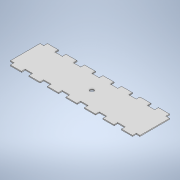
# Autodesk Inventor part: BridgeBottom
Saved by Autodesk Inventor 2022 (Build 260153000, 153)
## iProperties
Created: 2022-03-02
Part Number: BridgeBottom
Material: Generic
Document SubType Name: Modeling
Designer: anjarwala7025
Density: 1 g/cm^3
Appearance: Default
Author: anjarwala7025
Autodesk Inventor part; units mm, degrees
ref_plane "YZ Plane" through (0, 0, 0) normal (1, 0, 0) x (0, 1, 0)
ref_plane "XZ Plane" through (0, 0, 0) normal (0, 1, 0) x (-1, 0, 0)
ref_plane "XY Plane" through (0, 0, 0) normal (0, 0, 1) x (1, 0, 0)
sketch "Sketch1" plane through (0, 0, 0) normal (0, 1, 0) x (-1, 0, 0)
  line L0 (0, 0) -> (-444.5, 0)
  line L1 (-444.5, 0) -> (-444.5, -127)
  line L2 (-444.5, -127) -> (0, -127)
  line L3 (0, -127) -> (0, 0)
  dimension "d0" = 444.5
  dimension "d1" = 127
  constraints: 8 end point, 2 parallel, 1 horizontal, 1 perpendicular
  measures "d0" distance of L2.end L1.end
  measures "d1" distance of L1.end L0.end
extrude "Extrusion1" add sketch "Sketch1" along normal blind 3.175
sketch "Sketch2" plane through (0, 3.175, 0) normal (0, 1, 0) x (1, 0, 0)
  line L0 (0, 127) -> (0, 0) projected
  line L1 (0, 114.3) -> (12.7, 114.3)
  line L2 (12.7, 114.3) -> (12.7, 127)
  line L3 (444.5, 127) -> (0, 127) projected
  line L4 (50.8, 127) -> (50.8, 114.3)
  line L5 (50.8, 114.3) -> (76.2, 114.3)
  line L6 (76.2, 114.3) -> (76.2, 127)
  line L7 (114.3, 127) -> (114.3, 114.3)
  line L8 (114.3, 114.3) -> (139.7, 114.3)
  line L9 (139.7, 114.3) -> (139.7, 127)
  line L10 (177.8, 127) -> (177.8, 114.3)
  line L11 (177.8, 114.3) -> (203.2, 114.3)
  line L12 (203.2, 114.3) -> (203.2, 127)
  line L13 (241.3, 127) -> (241.3, 114.3)
  line L14 (241.3, 114.3) -> (266.7, 114.3)
  line L15 (266.7, 114.3) -> (266.7, 127)
  line L16 (304.8, 127) -> (304.8, 114.3)
  line L17 (304.8, 114.3) -> (330.2, 114.3)
  line L18 (330.2, 114.3) -> (330.2, 127)
  line L19 (368.3, 127) -> (368.3, 114.3)
  line L20 (368.3, 114.3) -> (393.7, 114.3)
  line L21 (393.7, 114.3) -> (393.7, 127)
  line L22 (431.8, 127) -> (431.8, 114.3)
  line L23 (431.8, 114.3) -> (444.5, 114.3)
  line L24 (444.5, 0) -> (444.5, 127) projected
  line L25 (0, 114.3) -> (0, 127)
  line L26 (50.8, 127) -> (76.2, 127)
  line L27 (114.3, 127) -> (139.7, 127)
  line L28 (177.8, 127) -> (203.2, 127)
  line L29 (241.3, 127) -> (266.7, 127)
  line L30 (304.8, 127) -> (330.2, 127)
  line L31 (368.3, 127) -> (393.7, 127)
  line L32 (431.8, 127) -> (444.5, 127)
  line L33 (0, 127) -> (12.7, 127)
  point P0 (444.5, 114.3)
  point P1 (12.7, 127)
  dimension "d4" = 12.7
  dimension "d6" = 12.7
  dimension "d7" = 12.7
  dimension "d8" = 12.7
  dimension "d9" = 25.4
  dimension "d10" = 38.1
  dimension "d11" = 25.4
  dimension "d12" = 38.1
  dimension "d13" = 25.4
  dimension "d14" = 38.1
  dimension "d15" = 25.4
  dimension "d16" = 38.1
  dimension "d17" = 25.4
  dimension "d18" = 38.1
  dimension "d19" = 25.4
  dimension "d20" = 38.1
  dimension "d22" = 0
  dimension "d42" = 12.7
  dimension "d53" = 38.1
  constraints: 62 end point, 13 vertical, 9 perpendicular, 7 horizontal, 1 collinear, 1 point on line, 14 other
  measures "d4" distance of L1.start L1.end
  measures "d6" length of L1
  measures "d7" distance of L1.end L2.end
  measures "d8" distance of L4.start L4.end
  measures "d9" distance of L4.end L5.end
  measures "d10" distance between parallel lines of L4 L2
  measures "d11" distance of L7.end L8.end
  measures "d12" distance between parallel lines of L7 L6
  measures "d13" distance of L10.end L11.end
  measures "d14" distance between parallel lines of L10 L9
  measures "d15" distance of L13.end L14.end
  measures "d16" distance between parallel lines of L13 L12
  measures "d17" distance of L16.end L17.end
  measures "d18" distance between parallel lines of L16 L15
  measures "d19" distance of L19.end L20.end
  measures "d20" distance between parallel lines of L19 L18
  measures "d22" distance from line of L24 L23.end
  measures "d42" distance of L22.start L22.end
  measures "d53" distance between parallel lines of L22 L21
extrude "Extrusion2" cut sketch "Sketch2" against normal through all
sketch "Sketch3" plane through (0, 3.175, 0) normal (0, 1, 0) x (1, 0, 0)
  line L0 (0, 0) -> (444.5, 0) projected
  line L1 (0, 0) -> (12.7, 0)
  line L2 (12.7, 0) -> (12.7, 12.7)
  line L3 (12.7, 12.7) -> (0, 12.7)
  line L4 (0, 12.7) -> (0, 0)
  line L5 (50.8, 0) -> (76.2, 0)
  line L6 (76.2, 0) -> (76.2, 12.7)
  line L7 (76.2, 12.7) -> (50.8, 12.7)
  line L8 (50.8, 12.7) -> (50.8, 0)
  line L9 (114.3, 0) -> (139.7, 0)
  line L10 (139.7, 0) -> (139.7, 12.7)
  line L11 (139.7, 12.7) -> (114.3, 12.7)
  line L12 (114.3, 12.7) -> (114.3, 0)
  line L13 (177.8, 0) -> (203.2, 0)
  line L14 (203.2, 0) -> (203.2, 12.7)
  line L15 (203.2, 12.7) -> (177.8, 12.7)
  line L16 (177.8, 12.7) -> (177.8, 0)
  line L17 (241.3, 0) -> (266.7, 0)
  line L18 (266.7, 0) -> (266.7, 12.7)
  line L19 (266.7, 12.7) -> (241.3, 12.7)
  line L20 (241.3, 12.7) -> (241.3, 0)
  line L21 (304.8, 0) -> (330.2, 0)
  line L22 (330.2, 0) -> (330.2, 12.7)
  line L23 (330.2, 12.7) -> (304.8, 12.7)
  line L24 (304.8, 12.7) -> (304.8, 0)
  line L25 (368.3, 0) -> (393.7, 0)
  line L26 (393.7, 0) -> (393.7, 12.7)
  line L27 (393.7, 12.7) -> (368.3, 12.7)
  line L28 (368.3, 12.7) -> (368.3, 0)
  line L29 (444.5, 0) -> (444.5, 114.3) projected
  line L30 (444.5, 0) -> (431.8, 0)
  line L31 (431.8, 0) -> (431.8, 12.7)
  line L32 (431.8, 12.7) -> (444.5, 12.7)
  line L33 (444.5, 12.7) -> (444.5, 0)
  point P0 (431.8, 0)
  point P1 (393.7, 0)
  point P2 (330.2, 0)
  point P3 (266.7, 0)
  point P4 (203.2, 0)
  point P5 (139.7, 0)
  point P6 (50.8, 0)
  point P7 (76.2, 0)
  point P8 (12.7, 0)
  dimension "d25" = 12.7
  dimension "d26" = 12.7
  dimension "d27" = 25.4
  dimension "d28" = 38.1
  dimension "d29" = 25.4
  dimension "d30" = 25.4
  dimension "d31" = 25.4
  dimension "d32" = 25.4
  dimension "d33" = 25.4
  dimension "d34" = 12.7
  dimension "d35" = 38.1
  dimension "d36" = 38.1
  dimension "d37" = 38.1
  dimension "d38" = 38.1
  dimension "d39" = 38.1
  constraints: 64 end point, 16 parallel, 11 point on line, 8 horizontal, 8 perpendicular
  measures "d25" distance of L3.end L2.end
  measures "d26" distance of L2.end L1.end
  measures "d27" distance of L7.end L6.end
  measures "d28" distance between parallel lines of L8 L2
  measures "d29" distance of L11.end L10.end
  measures "d30" distance of L15.end L14.end
  measures "d31" distance of L19.end L18.end
  measures "d32" distance of L23.end L22.end
  measures "d33" distance of L27.end L26.end
  measures "d34" distance of L31.end L32.end
  measures "d35" distance between parallel lines of L12 L6
  measures "d36" distance between parallel lines of L16 L10
  measures "d37" distance between parallel lines of L20 L14
  measures "d38" distance between parallel lines of L24 L18
  measures "d39" distance between parallel lines of L28 L22
extrude "Extrusion3" cut sketch "Sketch3" against normal through all
sketch "Sketch4" plane through (0, 3.175, 0) normal (0, 1, 0) x (1, 0, 0)
  circle A0 centre (228.6, 63.5) radius 6.35
  line L0 (0, 114.3) -> (0, 12.7) projected
  line L1 (241.3, 127) -> (203.2, 127) projected
  point P0 (0, 0)
  dimension "d43" = 12.7
  dimension "d44" = 228.6
  dimension "d45" = 63.5
  constraints: 1 centre point
  measures "d43" diameter of A0
  measures "d44" distance from line of A0.centre L0
  measures "d45" distance from line of A0.centre L1
hole "Hole1" at (228.6, 3.175, -63.5) direction (0, -1, 0) diameter 12.7 end through all
body "Solid1"
